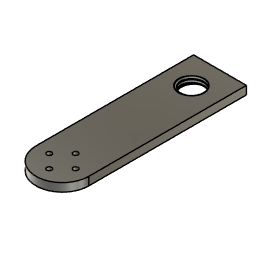
_Arm limb 2.1a77d3d6-5606-4075-9069-15030fea9f4f (Autodesk Fusion 360 design; units mm, degrees)
Autodesk Fusion 360 part; units mm, degrees
note: some values were not read from the file. Chosen so that the rebuilt part matches the saved one: which face or edge a step refers to; where a thread starts.
sketch "Sketch1" plane through (0, 0, 0) normal (0, 0, 1) x (1, 0, 0)
  line L0 (0, 95.5) -> (32, 95.5)
  line L1 (32, 95.5) -> (32, 0)
  line L2 (32, 0) -> (0, 0)
  line L3 (0, 0) -> (0, 95.5)
  dimension "d1" = 32
  dimension "d2" = 95.5
  constraint horizontal L0
  constraint vertical L1
  constraint horizontal L2
  constraint vertical L3
  measures "d1" distance of L0.start L0.end
  measures "d2" distance of L0.start L2.end
extrude "Extrude1" add sketch "Sketch1" along normal blind 5
sketch "Sketch2" plane through (0, 0, 0) normal (0, 0, 1) x (1, 0, 0)
  circle A0 centre (16, 0) radius 16
  dimension "d5" = 32
  measures "d5" diameter of A0
extrude "Extrude2" add sketch "Sketch2" along normal blind 5
sketch "Sketch3" plane through (0, 0, 5) normal (0, 0, 1) x (-1, 0, 0)
  line L0 (-32, 0) -> (-32, -95.5)
  line L1 (-32, -95.5) -> (0, -95.5)
  line L2 (0, -95.5) -> (0, 0)
  arc A0 (0, 0) -> (-32, 0) centre (-16, 0) ccw
  circle A1 centre (-16, 8) radius 1.5
  circle A2 centre (-8, 0) radius 1.5
  circle A3 centre (-16, -8) radius 1.5
  circle A4 centre (-24, 0) radius 1.5
  dimension "d8" = 3
  dimension "d9" = 3
  dimension "d10" = 3
  dimension "d11" = 3
  measures "d8" diameter of A1
  measures "d9" diameter of A2
  measures "d10" diameter of A3
  measures "d11" diameter of A4
extrude "Extrude3" cut sketch "Sketch3" against normal blind 5 contours A1 | A2 | A3 | A4
hole "Hole1" at (15.6649, 79.2961, 5) direction (0, 0, -1) diameter 14.023 depth 25 tip angle 118
thread "Thread1" "ISO Metric profile 16.0 M16x2 6H" major diameter 16.2505 minor diameter 14.0225 pitch 2 angle 60 modelled right hand crest width 0.5471 on face at (16.0144, 72.2933, 3.3333) crest through (15.6649, 72.2849, 0)
